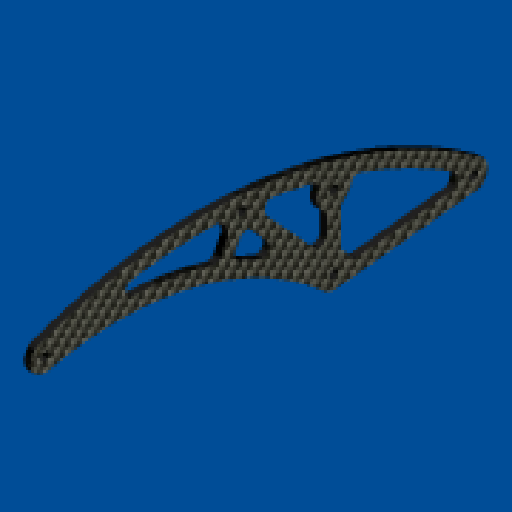
# Autodesk Inventor part: upperArmHanger
Saved by Autodesk Inventor 2023 (Build 270158030, 158C)
## iProperties
Created: 2023-03-03
Part Number: upperArmHanger
Material: CFRP
Document SubType Name: Modeling
Designer: kumpu
Density: 1.43 g/cm^3
Appearance: Glossy - Black
Author: kumpu
Autodesk Inventor part; units mm, degrees
ref_plane "YZ Plane" through (0, 0, 0) normal (1, 0, 0) x (0, 1, 0)
ref_plane "XZ Plane" through (0, 0, 0) normal (0, 1, 0) x (-1, 0, 0)
ref_plane "XY Plane" through (0, 0, 0) normal (0, 0, 1) x (1, 0, 0)
sketch "Sketch1" plane through (0, 0, 0) normal (1, 0, 0) x (0, 1, 0)
  circle A0 centre (0, 0) radius 13.462
  circle A1 centre (16.5768, -125.9135) radius 2
  line L0 (16.5768, -125.9135) -> (0, 0) construction
  circle A2 centre (0, 0) radius 35 construction
  circle A3 centre (10, -64.4908) radius 2 projected
  circle A4 centre (42, -64.4908) radius 2 projected
  circle A5 centre (54, -23.9908) radius 2 projected
  circle A6 centre (42, 62.5092) radius 2 projected
  line L1 (42, -64.4908) -> (10, -64.4908) construction
  line L2 (10.2629, -126.5896) -> (3.6861, -65.1669)
  arc A7 (10.2629, -126.5896) -> (21.7307, -129.623) centre (16.5768, -125.9135) ccw
  arc A8 (47.9527, 64.7201) -> (35.8225, 61.0392) centre (42, 62.5092) ccw
  circle A9 centre (54, -23.9908) radius 6.35 construction
  arc A10 (5.2567, -60.269) -> (3.6861, -65.1669) centre (10, -64.4908) ccw
  arc A11 (5.2567, -60.269) -> (35.8225, 61.0392) centre (-95.8375, 29.7084) ccw
  arc A12 (21.7307, -129.623) -> (47.9527, 64.7201) centre (-147.4509, -7.8554) ccw
  line L3 (10, -64.4908) -> (42, 62.5092) construction
  line L4 (42, 62.5092) -> (54, -23.9908) construction
  line L5 (54, -23.9908) -> (10, -64.4908) construction
  line L6 (42, -64.4908) -> (54, -23.9908) construction
  line L7 (16.5768, -125.9135) -> (10, -64.4908) construction
  line L8 (16.5768, -125.9135) -> (42, -64.4908) construction
  line L9 (54, -23.9908) -> (0, 0) construction
  arc A13 (20.9108, -119.646) -> (44.2744, -71.7635) centre (-147.4509, -7.8554) ccw
  arc A14 (35.073, -67.6658) -> (44.2744, -71.7635) centre (42, -64.4908) ccw
  arc A15 (10.8113, -72.0675) -> (16.927, -67.6658) centre (10, -64.4908) ccw
  arc A16 (20.9108, -119.646) -> (15.7656, -118.3368) centre (16.5768, -125.9135) ccw
  line L10 (15.7656, -118.3368) -> (10.8113, -72.0675)
  line L11 (16.927, -67.6658) -> (35.073, -67.6658)
  line L12 (35.073, -61.3158) -> (18.1375, -61.3158)
  arc A17 (47.8927, -59.6596) -> (35.073, -61.3158) centre (42, -64.4908) ccw
  arc A18 (47.8927, -59.6596) -> (53.2485, -31.5736) centre (-147.4509, -7.8554) ccw
  arc A19 (51.0536, -31.0181) -> (53.2485, -31.5736) centre (54, -23.9908) ccw
  line L13 (18.1375, -61.3158) -> (51.0536, -31.0181)
  line L14 (21.7098, -49.3972) -> (46.7531, -26.346)
  line L15 (46.3805, -24.0799) -> (36.8936, -19.8651)
  line L16 (48.9587, -18.2768) -> (38.9882, -13.8472)
  arc A20 (21.7098, -49.3972) -> (36.8936, -19.8651) centre (-95.8375, 29.7084) ccw
  arc A21 (54.4651, -16.385) -> (52.044, 24.4652) centre (-147.4509, -7.8554) ccw
  arc A22 (52.044, 24.4652) -> (45.7373, 24.0835) centre (48.9098, 23.9575) ccw
  arc A23 (38.9882, -13.8472) -> (45.7373, 24.0835) centre (-95.8375, 29.7084) ccw
  arc A24 (16.5768, -125.9135) -> (42, 62.5092) centre (-147.4509, -7.8554) ccw construction
  circle A25 centre (10, -64.4908) radius 3.175 construction
  circle A26 centre (54, -23.9908) radius 3.175 construction
  arc A27 (46.3805, -24.0799) -> (46.7531, -26.346) centre (54, -23.9908) ccw
  arc A28 (54.4651, -16.385) -> (48.9587, -18.2768) centre (54, -23.9908) ccw
  dimension "d0" = 26.924
  dimension "d1" = 4
  dimension "d2" = 70
  dimension "d3" = 127
  dimension "d4" = 82.5
  dimension "d5" = 6.35
  dimension "d6" = 6.35
  dimension "d7" = 7.62
  dimension "d8" = 3.175
  constraints: 40 point on circle, 34 end point, 25 centre point, 18 concentric, 17 tangent, 14 equal radius, 4 parallel, 3 coincident, 2 horizontal, 1 collinear
  measures "d0" diameter of A0
  measures "d1" diameter of A1
  measures "d2" diameter of A2
  measures "d3" distance of L0.start L0.end
  measures "d4" angle of L0 L1
  measures "d5" radius of A8
  measures "d6" diameter of A25
  measures "d7" radius of A17
  measures "d8" radius of A22
extrude "Extrusion1" add sketch "Sketch1" along normal blind 3 contours L2 A10 A11 A8 A12 A7
fillet "Fillet1" radius 3.175 18 edges at (1.5, 15.7656, -118.3368) (1.5, 10.8113, -72.0675) (1.5, 20.9108, -119.646) (1.5, 44.2744, -71.7635) (1.5, 35.073, -67.6658) (1.5, 16.927, -67.6658) (1.5, 47.8927, -59.6596) (1.5, 35.073, -61.3158) (1.5, 53.2485, -31.5736) (1.5, 51.0536, -31.0181) (1.5, 18.1375, -61.3158) (1.5, 46.3805, -24.0799) (1.5, 46.7531, -26.346) (1.5, 36.8936, -19.8651) (1.5, 21.7098, -49.3972) (1.5, 54.4651, -16.385) (1.5, 48.9587, -18.2768) (1.5, 38.9882, -13.8472)
body "Solid1"
